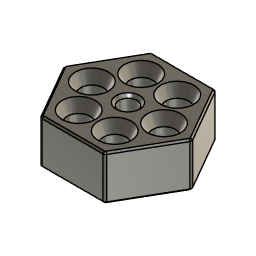
shaft_adapter_v2 (Autodesk Fusion 360 design; units mm, degrees)
Autodesk Fusion 360 part; units mm, degrees
sketch "Sketch1" plane through (0, 0, 0) normal (0, 0, 1) x (1, 0, 0)
  line L0 (-5.7735, 10) -> (-11.547, 0)
  line L1 (-11.547, 0) -> (-5.7735, -10)
  line L2 (-5.7735, -10) -> (5.7735, -10)
  line L3 (5.7735, -10) -> (11.547, 0)
  line L4 (11.547, 0) -> (5.7735, 10)
  line L5 (5.7735, 10) -> (-5.7735, 10)
  circle A0 centre (0, 0) radius 1.625
  circle A1 centre (-3.25, 5.6292) radius 2.05
  line L6 (0, 0) -> (-5.7735, 10) construction
  circle A2 centre (-6.5, 0) radius 2.05
  circle A3 centre (-3.25, -5.6292) radius 2.05
  circle A4 centre (3.25, -5.6292) radius 2.05
  circle A5 centre (6.5, 0) radius 2.05
  circle A6 centre (3.25, 5.6292) radius 2.05
  circle A7 centre (0, 0) radius 6.5 construction
  dimension "d1" = 10
  dimension "d2" = 3.25
  dimension "d4" = 4.1
  dimension "d9" = 360
  dimension "d10" = 13
  constraint coincident A0.centre L6.start
  constraint horizontal L5
  constraint coincident A1.centre L6
  constraint coincident A1.centre A7
  measures "d1" distance of A0.centre L5
  measures "d2" diameter of A0
  measures "d4" diameter of A1
  measures "d10" diameter of A7
extrude "Extrude1" add sketch "Sketch1" along normal blind 8
chamfer "Chamfer3" distance 0.5 angle 45 1 edges at (-1.515, 0.5876, 0)
chamfer "Chamfer3" distance 0.5 angle 45 1 edges at (-1.515, 0.5876, 8)
fillet "Fillet1" radius 0.5 6 edges at (-5.7735, -10, 4) (5.7735, -10, 4) (11.547, 0, 4) (5.7735, 10, 4) (-5.7735, 10, 4) (-11.547, 0, 4)
chamfer "Chamfer4" distance 0.3 angle 45 24 edges at (0, -10, 8) (5.7348, -9.933, 8) (8.6603, -5, 8) (11.4697, 0, 8) (8.6603, 5, 8) (5.7348, 9.933, 8) (0, 10, 8) (-5.7348, 9.933, 8) (-8.6603, 5, 8) (-11.4697, 0, 8) (-8.6603, -5, 8) (-5.7348, -9.933, 8) (0, -10, 0) (5.7348, -9.933, 0) (8.6603, -5, 0) (11.4697, 0, 0) (8.6603, 5, 0) (5.7348, 9.933, 0) (0, 10, 0) (-5.7348, 9.933, 0) (-8.6603, 5, 0) (-11.4697, 0, 0) (-8.6603, -5, 0) (-5.7348, -9.933, 0)
chamfer "Chamfer2" distance 2 angle 25 6 edges at (1.3387, 6.3705, 8) (-5.1613, 6.3705, 8) (-8.4113, 0.7413, 8) (-5.1613, -4.8879, 8) (1.3387, -4.8879, 8) (4.5887, 0.7413, 8) measured on face at (5.2975, 5.527, 5.3333) measured on face at (-1.2025, 5.527, 5.3333) measured on face at (-4.4525, -0.1022, 5.3333) measured on face at (-1.2025, -5.7313, 5.3333) measured on face at (5.2975, -5.7313, 5.3333) measured on face at (8.5475, -0.1022, 5.3333)
chamfer "Chamfer5" distance 2 angle 25 6 edges at (-5.1613, -4.8879, 0) (1.3387, -4.8879, 0) (4.5887, 0.7413, 0) (1.3387, 6.3705, 0) (-5.1613, 6.3705, 0) (-8.4113, 0.7413, 0) measured on face at (-1.2102, -5.8333, 2) measured on face at (5.2898, -5.8333, 2) measured on face at (8.5398, -0.2041, 2) measured on face at (5.2898, 5.4251, 2) measured on face at (-1.2102, 5.4251, 2) measured on face at (-4.4602, -0.2041, 2)
named bodies: "Shaft_adapter"
